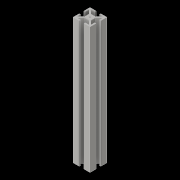
# Autodesk Inventor part: ProfileTwo
Saved by Autodesk Inventor 2016 (Build 200138000, 138)
## iProperties
Created: 2017-01-21
Part Number: ProfileTwo
Material: Generic
Document SubType Name: Modeling
Designer: Alexis Renderos
Density: 1 g/cm^3
Appearance: Default
Author: Alexis Renderos
Autodesk Inventor part; units mm, degrees
ref_plane "YZ Plane" through (0, 0, 0) normal (1, 0, 0) x (0, 1, 0)
ref_plane "XZ Plane" through (0, 0, 0) normal (0, 1, 0) x (-1, 0, 0)
ref_plane "XY Plane" through (0, 0, 0) normal (0, 0, 1) x (1, 0, 0)
sketch "Sketch1" plane through (0, 0, 0) normal (0, 1, 0) x (-1, 0, 0)
  line L0 (0, -29.8704) -> (0, 29.8704) projected
  line L1 (-29.8704, 0) -> (29.8704, 0) projected
  line L2 (0, -21.336) -> (0, 21.336)
  line L3 (-21.336, 0) -> (21.336, 0)
  line L4 (15.24, -15.24) -> (4.191, -15.24)
  line L5 (-15.24, -15.24) -> (-4.191, -15.24)
  line L6 (15.24, 4.191) -> (12.827, 4.191)
  line L7 (12.827, -4.191) -> (15.24, -4.191)
  line L8 (-4.191, 12.827) -> (-4.191, 15.24)
  line L9 (4.191, 15.24) -> (4.191, 12.827)
  line L10 (-11.1208, -12.827) -> (-4.212, -5.9182)
  line L11 (-12.827, -11.1208) -> (-5.9182, -4.212)
  line L12 (-5.9182, 4.212) -> (-12.827, 11.1208)
  line L13 (-4.212, 5.9182) -> (-11.1208, 12.827)
  line L14 (-1.7062, 0) -> (0, 1.7062)
  line L15 (4.212, 5.9182) -> (11.1208, 12.827)
  line L16 (0, -1.7062) -> (1.7062, 0)
  line L17 (5.9182, 4.212) -> (12.827, 11.1208)
  line L18 (12.827, -11.1208) -> (5.9182, -4.212)
  line L19 (1.7062, 0) -> (0, 1.7062)
  line L20 (11.1208, -12.827) -> (4.212, -5.9182)
  line L21 (0, -1.7062) -> (-1.7062, 0)
  line L22 (4.191, -12.827) -> (4.191, -15.24)
  line L23 (-15.24, 4.191) -> (-12.827, 4.191)
  line L24 (-4.191, -15.24) -> (-4.191, -12.827)
  line L25 (-12.827, -4.191) -> (-15.24, -4.191)
  line L26 (11.1208, 12.827) -> (4.191, 12.827)
  line L27 (-4.191, 12.827) -> (-11.1208, 12.827)
  line L28 (-12.827, 11.1208) -> (-12.827, 4.191)
  line L29 (-12.827, -4.191) -> (-12.827, -11.1208)
  line L30 (-11.1208, -12.827) -> (-4.191, -12.827)
  line L31 (4.191, -12.827) -> (11.1208, -12.827)
  line L32 (12.827, -11.1208) -> (12.827, -4.191)
  line L33 (12.827, 4.191) -> (12.827, 11.1208)
  line L34 (-15.24, -15.24) -> (-15.24, -4.191)
  line L35 (-15.24, 4.191) -> (-15.24, 15.24)
  line L36 (15.24, -15.24) -> (4.191, -15.24)
  line L37 (-4.191, -15.24) -> (-15.24, -15.24)
  line L38 (15.24, 15.24) -> (15.24, 4.191)
  line L39 (15.24, -4.191) -> (15.24, -15.24)
  line L40 (-15.24, 15.24) -> (-4.191, 15.24)
  line L41 (4.191, 15.24) -> (15.24, 15.24)
  line L42 (4.212, 5.9182) -> (-4.212, 5.9182)
  line L43 (-5.9182, 4.212) -> (-5.9182, -4.212)
  line L44 (-4.212, -5.9182) -> (4.212, -5.9182)
  line L45 (5.9182, -4.212) -> (5.9182, 4.212)
  line L46 (5.9182, 5.9182) -> (-5.9182, -5.9182) construction
  line L47 (-5.9182, 5.9182) -> (5.9182, -5.9182) construction
  point P0 (0, 0)
  point P1 (0, 0)
  point P2 (0, -4.191)
  point P3 (-4.191, 0)
  point P4 (0, 4.191)
  point P5 (4.191, 0)
  dimension "d0" = 11.049
  dimension "d1" = 30.48
  dimension "d2" = 30.48
  dimension "d3" = 11.8364
  dimension "d4" = 11.8364
  constraints: 92 end point, 22 parallel, 9 perpendicular, 8 point on line, 4 horizontal, 2 midpoint, 1 collinear
  measures "d0" distance of L5.end L5.start
  measures "d1" distance of L34.start L35.end
  measures "d2" distance of L35.end L38.start
  measures "d3" distance of L47.end L46.end
  measures "d4" distance of L46.end L47.start
extrude "Extrusion1" add sketch "Sketch1" along normal blind 228.6 contours L44 L10 L30 L24 L5 L34 L25 L29 L11 L43 L1 L21 L0 | L0 L16 L1 L45 L18 L32 L7 L39 L4 L22 L31 L20 L44 | L19 L0 L42 L15 L26 L9 L41 L38 L6 L33 L17 L45 L1 | L1 L43 L12 L28 L23 L35 L40 L8 L27 L13 L42 L0 L14
body "Solid1"
